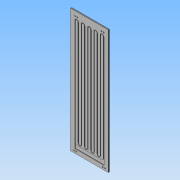
# Autodesk Inventor part: Ply back
Saved by Autodesk Inventor 2013 (Build 170138000, 138)
## iProperties
Created: 2018-07-07
Part Number: Ply back
Material: Generic
Document SubType Name: Modeling
Designer: Jeff Vyduna
Density: 1 g/cm^3
Author: Jeff Vyduna
Autodesk Inventor part; units mm, degrees
ref_plane "YZ Plane" through (0, 0, 0) normal (1, 0, 0) x (0, 1, 0)
ref_plane "XZ Plane" through (0, 0, 0) normal (0, 1, 0) x (-1, 0, 0)
ref_plane "XY Plane" through (0, 0, 0) normal (0, 0, 1) x (1, 0, 0)
sketch "TwoLineColumn" plane through (0, 0, 0) normal (0, 0, 1) x (1, 0, 0)
  line L0 (50.8, -753.9609) -> (50.8, 922.4391) construction
  line L1 (101.6, -753.9609) -> (101.6, 922.4391) construction
  arc A0 (101.6, 922.4391) -> (50.8, 922.4391) centre (76.2, 922.4391) ccw construction
  arc A1 (101.6, -753.9609) -> (152.4, -753.9609) centre (127, -753.9609) ccw construction
  line L2 (56.896, -753.9609) -> (56.896, 922.4391)
  arc A2 (95.504, 922.4391) -> (56.896, 922.4391) centre (76.2, 922.4391) ccw
  line L3 (95.504, 922.4391) -> (95.504, -753.9609)
  arc A3 (95.504, -753.9609) -> (158.496, -753.9609) centre (127, -753.9609) ccw
  line L4 (44.704, -753.9609) -> (44.704, 922.4391)
  arc A4 (107.696, 922.4391) -> (44.704, 922.4391) centre (76.2, 922.4391) ccw
  line L5 (107.696, 922.4391) -> (107.696, -753.9609)
  arc A5 (107.696, -753.9609) -> (146.304, -753.9609) centre (127, -753.9609) ccw
  line L6 (50.8, -753.9609) -> (152.4, -753.9609) construction
  dimension "d4" = 1676.4
  dimension "lineSpacing" = 50.8
  dimension "d6" = 25.4
  dimension "d9" = 6.096
  dimension "d10" = 6.096
  measures "d4" distance of L0.start L0.end
  measures "lineSpacing" distance between parallel lines of L1 L0
  measures "d6" radius of A1
  measures "d9" distance between parallel lines of L1 L3
  measures "d10" distance between parallel lines of L5 L1
sketch "TwoLineColumnEnd" plane through (0, 0, 0) normal (0, 0, 1) x (1, 0, 0)
  line L0 (103.0524, -945.1843) -> (103.0524, 731.2157)
  arc A0 (166.0444, 731.2157) -> (103.0524, 731.2157) centre (134.5484, 731.2157) ccw
  line L1 (166.0444, 731.2157) -> (166.0444, -945.1843)
  line L2 (109.1484, -945.1843) -> (109.1484, 731.2157) construction
  line L3 (159.9484, -945.1843) -> (159.9484, 731.2157) construction
  arc A1 (159.9484, 731.2157) -> (109.1484, 731.2157) centre (134.5484, 731.2157) ccw construction
  line L4 (115.2444, -945.1843) -> (115.2444, 731.2157)
  arc A2 (153.8524, 731.2157) -> (115.2444, 731.2157) centre (134.5484, 731.2157) ccw
  line L5 (153.8524, 731.2157) -> (153.8524, -945.1843)
  line L6 (109.1484, -945.1843) -> (159.9484, -945.1843) construction
  dimension "d22" = 1676.4
  dimension "d23" = 50.8
  dimension "d25" = 6.096
  dimension "d26" = 6.096
  dimension "d29" = 50.8
  measures "d22" distance of L2.start L2.end
  measures "d23" distance between parallel lines of L3 L2
  measures "d25" distance between parallel lines of L3 L5
  measures "d26" distance between parallel lines of L1 L3
  measures "d29" distance of L2.start L6.end
sketch "15mm Neon profile" plane through (0, 0, 0) normal (0, 0, 1) x (1, 0, 0)
  circle A0 centre (522.6685, 24.7098) radius 6.985 construction
  line L0 (516.6995, 21.082) -> (528.6375, 21.082) construction
  line L1 (528.6375, 21.082) -> (528.6375, 6.35) construction
  line L2 (528.6375, 6.35) -> (516.6995, 6.35) construction
  line L3 (516.6995, 6.35) -> (516.6995, 21.082) construction
  point P0 (522.6685, 16.011)
  dimension "d73" = 13.97
  dimension "d74" = 11.938
  dimension "d76" = 14.732
  measures "d73" diameter of A0
  measures "d74" distance of L0.start L0.end
  measures "d76" distance of L0.end L1.end
sketch "U Bolt hole and bore" plane through (0, 0, 0) normal (0, 0, 1) x (1, 0, 0)
  circle A0 centre (40.0435, 30.4025) radius 9.525
  circle A1 centre (74.9685, 30.4025) radius 9.525
  circle A2 centre (40.0435, 30.4025) radius 3.9688
  circle A3 centre (74.9685, 30.4025) radius 3.9688
  point P0 (68.2625, 33.02)
  dimension "d100" = 19.05
  dimension "d102" = 34.925
  dimension "d105" = 7.9375
  measures "d100" diameter of A0
  measures "d102" distance of A1.centre A0.centre
  measures "d105" diameter of A2
sketch "Stock" plane through (0, 0, 0) normal (0, 0, 1) x (1, 0, 0)
  line L0 (0, 0) -> (604.8375, 0)
  line L1 (604.8375, 0) -> (604.8375, 1981.2)
  line L2 (604.8375, 1981.2) -> (0, 1981.2)
  line L3 (0, 1981.2) -> (0, 0)
  dimension "d1" = 604.8375
  dimension "d2" = 1981.2
  constraints: 8 end point, 2 parallel, 1 coincident, 1 horizontal, 1 perpendicular
  measures "d1" distance of L2.end L1.end
  measures "d2" distance of L1.end L0.end
extrude "Stck Extrusion" add sketch "Stock" along normal blind 19.05
sketch "LEDPocket" plane through (0, 0, 19.05) normal (0, 0, 1) x (1, 0, 0)
  line L0 (0, 0) -> (604.8375, 0) projected
  line L1 (604.8375, 0) -> (604.8375, 1981.2) projected
  line L2 (63.5, 1981.2) -> (63.5, 0) construction
  line L3 (541.3375, 1981.2) -> (541.3375, 0) construction
  line L4 (67.7228, 171.196) -> (67.7228, 68.2625)
  line L5 (72.4853, 63.5) -> (532.3523, 63.5)
  line L6 (537.1148, 68.2625) -> (537.1147, 171.196)
  line L7 (79.9148, 171.196) -> (79.9148, 152.4)
  line L8 (105.3148, 127) -> (499.5227, 127)
  line L9 (524.9227, 152.4) -> (524.9227, 171.196)
  arc A0 (79.9148, 152.4) -> (105.3148, 127) centre (105.3148, 152.4) ccw
  arc A1 (499.5227, 127) -> (524.9227, 152.4) centre (499.5227, 152.4) ccw
  arc A2 (67.7228, 68.2625) -> (72.4853, 63.5) centre (72.4853, 68.2625) ccw
  arc A3 (532.3523, 63.5) -> (537.1148, 68.2625) centre (532.3523, 68.2625) ccw
  line L10 (474.1228, 171.196) -> (474.1227, 1847.596)
  arc A4 (537.1147, 1847.596) -> (474.1227, 1847.596) centre (505.6187, 1847.596) ccw
  line L11 (537.1147, 1847.596) -> (537.1147, 171.196)
  line L12 (480.2188, 171.196) -> (480.2188, 1847.596) construction
  line L13 (531.0187, 171.196) -> (531.0187, 1847.596) construction
  arc A5 (531.0187, 1847.596) -> (480.2188, 1847.596) centre (505.6187, 1847.596) ccw construction
  line L14 (486.3148, 171.196) -> (486.3148, 1847.596)
  arc A6 (524.9227, 1847.596) -> (486.3148, 1847.596) centre (505.6187, 1847.596) ccw
  line L15 (524.9227, 1847.596) -> (524.9227, 171.196)
  line L16 (480.2188, 171.196) -> (531.0187, 171.196) construction
  line L17 (67.7228, 171.196) -> (67.7228, 1847.596)
  arc A7 (130.7148, 1847.596) -> (67.7228, 1847.596) centre (99.2188, 1847.596) ccw
  line L18 (130.7148, 1847.596) -> (130.7148, 171.196)
  arc A8 (130.7148, 171.196) -> (169.3228, 171.196) centre (150.0188, 171.196) ccw
  line L19 (73.8188, 171.196) -> (73.8188, 1847.596) construction
  line L20 (124.6188, 171.196) -> (124.6188, 1847.596) construction
  arc A9 (124.6188, 1847.596) -> (73.8188, 1847.596) centre (99.2188, 1847.596) ccw construction
  arc A10 (124.6188, 171.196) -> (175.4188, 171.196) centre (150.0188, 171.196) ccw construction
  line L21 (79.9148, 171.196) -> (79.9148, 1847.596)
  arc A11 (118.5228, 1847.596) -> (79.9148, 1847.596) centre (99.2188, 1847.596) ccw
  line L22 (118.5228, 1847.596) -> (118.5228, 171.196)
  arc A12 (118.5228, 171.196) -> (181.5148, 171.196) centre (150.0188, 171.196) ccw
  line L23 (73.8188, 171.196) -> (175.4188, 171.196) construction
  line L24 (169.3228, 171.196) -> (169.3228, 1847.596)
  arc A13 (232.3148, 1847.596) -> (169.3228, 1847.596) centre (200.8187, 1847.596) ccw
  line L25 (232.3148, 1847.596) -> (232.3148, 171.196)
  arc A14 (232.3148, 171.196) -> (270.9228, 171.196) centre (251.6188, 171.196) ccw
  line L26 (175.4188, 171.196) -> (175.4188, 1847.596) construction
  line L27 (226.2188, 171.196) -> (226.2188, 1847.596) construction
  arc A15 (226.2188, 1847.596) -> (175.4188, 1847.596) centre (200.8187, 1847.596) ccw construction
  arc A16 (226.2188, 171.196) -> (277.0188, 171.196) centre (251.6188, 171.196) ccw construction
  line L28 (181.5148, 171.196) -> (181.5148, 1847.596)
  arc A17 (220.1228, 1847.596) -> (181.5148, 1847.596) centre (200.8187, 1847.596) ccw
  line L29 (220.1228, 1847.596) -> (220.1228, 171.196)
  arc A18 (220.1228, 171.196) -> (283.1148, 171.196) centre (251.6188, 171.196) ccw
  line L30 (270.9228, 171.196) -> (270.9228, 1847.596)
  arc A19 (333.9148, 1847.596) -> (270.9228, 1847.596) centre (302.4187, 1847.596) ccw
  line L31 (333.9148, 1847.596) -> (333.9148, 171.196)
  arc A20 (333.9148, 171.196) -> (372.5228, 171.196) centre (353.2188, 171.196) ccw
  line L32 (277.0188, 171.196) -> (277.0188, 1847.596) construction
  line L33 (327.8188, 171.196) -> (327.8188, 1847.596) construction
  arc A21 (327.8188, 1847.596) -> (277.0188, 1847.596) centre (302.4187, 1847.596) ccw construction
  arc A22 (327.8188, 171.196) -> (378.6188, 171.196) centre (353.2188, 171.196) ccw construction
  line L34 (283.1148, 171.196) -> (283.1148, 1847.596)
  arc A23 (321.7228, 1847.596) -> (283.1148, 1847.596) centre (302.4187, 1847.596) ccw
  line L35 (321.7228, 1847.596) -> (321.7228, 171.196)
  arc A24 (321.7228, 171.196) -> (384.7147, 171.196) centre (353.2188, 171.196) ccw
  line L36 (372.5228, 171.196) -> (372.5228, 1847.596)
  arc A25 (435.5148, 1847.596) -> (372.5228, 1847.596) centre (404.0188, 1847.596) ccw
  line L37 (435.5148, 1847.596) -> (435.5148, 171.196)
  arc A26 (435.5148, 171.196) -> (474.1228, 171.196) centre (454.8188, 171.196) ccw
  line L38 (378.6188, 171.196) -> (378.6188, 1847.596) construction
  line L39 (429.4188, 171.196) -> (429.4188, 1847.596) construction
  arc A27 (429.4188, 1847.596) -> (378.6188, 1847.596) centre (404.0188, 1847.596) ccw construction
  arc A28 (429.4188, 171.196) -> (480.2188, 171.196) centre (454.8188, 171.196) ccw construction
  line L40 (384.7147, 171.196) -> (384.7147, 1847.596)
  arc A29 (423.3228, 1847.596) -> (384.7147, 1847.596) centre (404.0188, 1847.596) ccw
  line L41 (423.3228, 1847.596) -> (423.3228, 171.196)
  arc A30 (423.3228, 171.196) -> (486.3148, 171.196) centre (454.8188, 171.196) ccw
  point P0 (0, 1981.2)
  point P1 (67.7228, 63.5)
  dimension "d7" = 73.8187
  dimension "d18" = 63.5
  dimension "d19" = 1981.2
  dimension "d20" = 1981.2
  dimension "d21" = 541.3375
  dimension "d31" = 63.5
  dimension "d32" = 63.5
  dimension "d33" = 44.196
  dimension "d34" = 25.4
  dimension "d35" = 4.7625
  dimension "d38" = 171.196
  dimension "d41" = 1676.4
  dimension "d42" = 50.8
  dimension "d43" = 6.096
  dimension "d44" = 6.096
  dimension "d45" = 50.8
  dimension "d49" = 1676.4
  dimension "d50" = 50.8
  dimension "d51" = 25.4
  dimension "d52" = 6.096
  dimension "d53" = 6.096
  dimension "d89" = 133.604
  constraints: 80 end point, 62 point on circle, 31 centre point, 31 tangent, 24 vertical, 22 parallel, 16 horizontal alignment, 8 equal radius, 5 perpendicular, 2 point on line, 1 coincident, 10 other
  measures "d7" distance from line of L19 point (0, 0)
  measures "d18" distance from line of point (0, 0) L2
  measures "d19" distance of L2.start L2.end
  measures "d20" distance of L3.start L3.end
  measures "d21" distance from line of L0.start L3
  measures "d31" vertical distance of L0.start point (67.723, 63.5)
  measures "d32" distance between parallel lines of L5 L8
  measures "d33" distance from line of L19.start L8
  measures "d34" radius of A0
  measures "d35" radius of A2
  measures "d38" distance from line of L19.start L0
  measures "d41" distance of L12.start L12.end
  measures "d42" distance between parallel lines of L13 L12
  measures "d43" distance between parallel lines of L13 L15
  measures "d44" distance between parallel lines of L11 L13
  measures "d45" distance of L12.start L16.end
  measures "d49" distance of L19.start L19.end
  measures "d50" distance between parallel lines of L20 L19
  measures "d51" radius of A10
  measures "d52" distance between parallel lines of L20 L22
  measures "d53" distance between parallel lines of L18 L20
  measures "d89" vertical distance of A7.centre point (0, 1981.2)
extrude "Extrusion3" cut sketch "LEDPocket" against normal blind 12.7
sketch "Side profile reference" plane through (0, 0, 0) normal (0, -1, 0) x (1, 0, 0)
  line L0 (0, 0) -> (604.8375, 0) projected
  line L1 (604.8375, 0) -> (604.8375, 19.05) projected
  line L2 (0, 19.05) -> (604.8375, 19.05) projected
  line L3 (0, 0) -> (0, 19.05) projected
  line L4 (598.4875, 38.1) -> (586.2955, 38.1) construction
  line L5 (586.2955, 38.1) -> (586.2955, 25.4) construction
  line L6 (586.2955, 25.4) -> (598.4875, 25.4) construction
  line L7 (598.4875, 25.4) -> (598.4875, 38.1) construction
  line L8 (604.8375, 19.05) -> (541.3375, 19.05) construction
  line L9 (541.3375, 19.05) -> (541.3375, 38.1) construction
  line L10 (541.3375, 38.1) -> (604.8375, 38.1) construction
  line L11 (604.8375, 38.1) -> (604.8375, 19.05) construction
  line L12 (547.6875, 38.1) -> (573.0875, 38.1) construction
  line L13 (573.0875, 38.1) -> (573.0875, 40.64) construction
  line L14 (573.0875, 40.64) -> (547.6875, 40.64) construction
  line L15 (547.6875, 40.64) -> (547.6875, 38.1) construction
  line L16 (579.4375, 40.64) -> (516.6995, 40.64) construction
  line L17 (516.6995, 40.64) -> (516.6995, 45.847) construction
  line L18 (516.6995, 45.847) -> (579.4375, 45.847) construction
  line L19 (579.4375, 45.847) -> (579.4375, 40.64) construction
  circle A0 centre (522.6685, 24.7098) radius 6.985 construction
  line L20 (516.6995, 21.082) -> (528.6375, 21.082) construction
  line L21 (528.6375, 21.082) -> (528.6375, 6.35) construction
  line L22 (528.6375, 6.35) -> (516.6995, 6.35) construction
  line L23 (516.6995, 6.35) -> (516.6995, 21.082) construction
  circle A1 centre (592.3915, 43.7598) radius 6.985 construction
  line L24 (586.4225, 40.132) -> (598.3605, 40.132) construction
  line L25 (598.3605, 40.132) -> (598.3605, 25.4) construction
  line L26 (598.3605, 25.4) -> (586.4225, 25.4) construction
  line L27 (586.4225, 25.4) -> (586.4225, 40.132) construction
  point P0 (566.7375, 19.05)
  point P1 (592.3915, 25.4)
  point P2 (592.3915, 25.4)
  dimension "d75" = 12.7
  dimension "d80" = 12.192
  dimension "d88" = 6.35
  dimension "d90" = 63.5
  dimension "d91" = 19.05
  dimension "d92" = 25.4
  dimension "d93" = 2.54
  dimension "d94" = 6.35
  dimension "d95" = 12.7
  dimension "d96" = 6.35
  dimension "d97" = 5.207
  dimension "d98" = 0
  dimension "d99" = 12.7
  constraints: 32 end point, 8 parallel, 5 horizontal, 4 perpendicular, 1 coincident, 1 collinear, 1 midpoint, 1 point on line, 1 other
  measures "d80" distance of L6.end L5.end
  measures "d88" horizontal distance of L1.end L6.end
  measures "d90" distance of L9.end L10.end
  measures "d91" distance of L8.end L9.end
  measures "d92" distance of L14.end L13.end
  measures "d93" distance of L13.end L12.end
  measures "d94" distance of L9.end L12.start
  measures "d96" horizontal distance of L16.start L12.end
  measures "d97" distance of L16.end L17.end
  measures "d99" vertical distance of L10.end L6.end
sketch "U-Bolt holes" plane through (0, 0, 19.05) normal (0, 0, 1) x (1, 0, 0)
  line L0 (0, 0) -> (604.8375, 0) projected
  line L1 (604.8375, 0) -> (604.8375, 1981.2) projected
  line L2 (0, 1981.2) -> (0, 0) projected
  line L3 (604.8375, 1981.2) -> (0, 1981.2) projected
  point P0 (53.975, 33.02)
  point P1 (88.9, 33.02)
  point P2 (515.9375, 33.02)
  point P3 (550.8625, 33.02)
  point P4 (531.8125, 1908.175)
  point P5 (496.8875, 1908.175)
  point P6 (73.025, 1908.175)
  point P7 (107.95, 1908.175)
  dimension "d109" = 33.02
  dimension "d110" = 34.925
  dimension "d111" = 34.925
  dimension "d112" = 19.05
  dimension "d113" = 53.975
  dimension "d114" = 53.975
  dimension "d115" = 34.925
  dimension "d116" = 34.925
  dimension "d117" = 19.05
  dimension "d126" = 73.025
  constraints: 6 horizontal alignment
  measures "d109" distance from line of L0 point (53.975, 33.02)
  measures "d110" distance of point (88.9, 33.02) point (53.975, 33.02)
  measures "d111" distance of point (550.862, 33.02) point (515.937, 33.02)
  measures "d112" horizontal distance of point (53.975, 33.02) point (73.025, 1908.175)
  measures "d113" distance from line of L1 point (550.862, 33.02)
  measures "d114" distance from line of L2 point (53.975, 33.02)
  measures "d115" distance of point (73.025, 1908.175) point (107.95, 1908.175)
  measures "d116" distance of point (531.812, 1908.175) point (496.887, 1908.175)
  measures "d117" horizontal distance of point (531.812, 1908.175) point (550.862, 33.02)
  measures "d126" distance from line of L3 point (73.025, 1908.175)
hole "Hole1" at (73.025, 1908.175, 19.05) at (107.95, 1908.175, 19.05) at (496.8875, 1908.175, 19.05) at (531.8125, 1908.175, 19.05) at (550.8625, 33.02, 19.05) at (515.9375, 33.02, 19.05) at (88.9, 33.02, 19.05) at (53.975, 33.02, 19.05) direction (0, 0, -1) diameter 7.9375 end through all counterbore diameter 19.05 counterbore depth 6.35
equation "\"d7\" = -4.5 * lineSpacing + 0.5 * signW"
equation "\"d18\" = borderW"
equation "\"d31\" = borderW"
equation "\"d4\" = litH"
equation "\"d6\" = 0.5 * lineSpacing"
equation "\"d9\" = 0.5 * pathW"
equation "\"d10\" = 0.5 * pathW"
equation "\"d22\" = litH"
equation "\"d25\" = 0.5 * pathW"
equation "\"d26\" = 0.5 * pathW"
equation "\"d29\" = lineSpacing"
equation "\"d1\" = signW"
equation "\"d2\" = signH"
equation "\"d19\" = signH"
equation "\"d20\" = signH"
equation "\"d21\" = signW - borderW"
equation "\"d32\" = ePocketH"
equation "\"d33\" = litHClearanceH"
equation "\"d34\" = minBendR"
equation "\"d35\" = 0.5 * pathEndMillD"
equation "\"d41\" = d46"
equation "\"d43\" = 0.5 * d48"
equation "\"d44\" = 0.5 * d48"
equation "\"d45\" = d47"
equation "\"d49\" = d54"
equation "\"d51\" = 0.5 * d50"
equation "\"d52\" = 0.5 * d55"
equation "\"d53\" = 0.5 * d55"
equation "\"litH\" = 1676.4"
equation "\"borderW\" = 63.5"
equation "\"pathEndMillD\" = 9.525"
equation "\"signW\" = -0.5 * pathEndMillD + 0.5 * ply4x8w"
equation "\"pathW\" = 12.192"
equation "\"ply4x8w\" = 1219.2"
equation "\"signH\" = 1981.2"
equation "\"borderPadding\" = 12.7"
equation "\"ePocketH\" = 63.5"
equation "\"minBendR\" = 25.4"
equation "\"d46\" = 1676.4"
equation "\"d48\" = 12.192"
equation "\"d54\" = 1676.4"
equation "\"d55\" = 12.192"
equation "\"litHClearanceH\" = 44.196"
equation "\"d47\" = 50.8"
body "Solid1"
